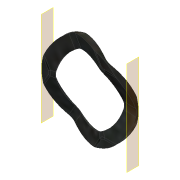
# Autodesk Inventor part: Nema 17 Sprung Washer
Saved by Autodesk Inventor 2020.2 (Build 242310000, 310)
## iProperties
Created: 2020-01-21
Part Number: Nema 17 Sprung Washer
Material: Steel
Document SubType Name: Modeling
Designer: james
Density: 7.85 g/cm^3
Appearance: Plate
Mass: 0.376842 g
Surface Area: 2.38464 cm^2
Volume: 0.0480053 cm^3
Author: james
Autodesk Inventor part; units mm, degrees
ref_plane "XZ Plane" through (0, 0, 0) normal (0, 1, 0) x (-1, 0, 0)
ref_plane "XY Plane" through (0, 0, 0) normal (0, 0, 1) x (1, 0, 0)
sketch "Sketch11" plane through (0, 0, 0) normal (0, 1, 0) x (-1, 0, 0)
  circle A0 centre (0, 0) radius 5.5
  circle A1 centre (0, 0) radius 7.75
  dimension "d82" = 11
  dimension "d83" = 15.5
  constraints: 2 centre point, 2 coincident
  measures "d82" diameter of A0
  measures "d83" diameter of A1
extrude "Extrusion7" add sketch "Sketch11" along normal blind 2
ref_plane "Work Plane6" through (7.75, 0, 0) normal (1, 0, 0) x (0, 1, 0)
sketch "Sketch14" plane through (7.75, 0, 0) normal (1, 0, 0) x (0, 1, 0)
  arc A0 (1.7, 0) -> (1.593716, 0.643303) centre (-0.3, 0) ccw
  line L0 (1.593716, 0.643303) -> (0.053142, 5.178348)
  line L1 (0, -7.75) -> (0, 7.75)
  arc A1 (0, 5.5) -> (0.053142, 5.178348) centre (1, 5.5) ccw
  line L2 (1.7, 0) -> (0, 0)
  line L3 (2, -7.75) -> (2, 7.75) construction
  line L4 (2, -5.5) -> (0, -5.5)
  line L5 (2, 5.5) -> (0, 5.5)
  point P0 (0, 7.75)
  dimension "d100" = 2
  dimension "d101" = 0.3
  dimension "d102" = 1
  constraints: 4 end point, 4 point on circle, 2 centre point, 2 tangent, 1 horizontal, 1 line through centre, 2 other
  measures "d100" radius of A0
  measures "d101" distance from line of L3 L2.start
  measures "d102" radius of A1
extrude "Extrusion10" cut sketch "Sketch14" against normal blind 7.75
mirror "Mirror5" about plane through (0, 0, 0) normal (0, 0, 1) of "Extrusion10"
pattern_circular "Circular Pattern2" count 3 over 360 about axis through (0, 0, 0) along (0, 1, 0) of "Extrusion10", "Mirror5"
ref_plane "Work Plane7" through (-7.75, 0, 0) normal (1, 0, 0) x (0, 1, 0)
sketch "Sketch15" plane through (-7.75, 0, 0) normal (1, 0, 0) x (0, 1, 0)
  line L0 (2, 5.5) -> (2, -5.5)
  line L1 (2, 0) -> (0.3, 0)
  arc A0 (2, -5.5) -> (1.946858, -5.178348) centre (1, -5.5) ccw
  arc A1 (0.3, 0) -> (0.406284, -0.643303) centre (2.3, 0) ccw
  line L2 (1.946858, -5.178348) -> (0.406284, -0.643303)
  point P0 (0, 0)
  dimension "d109" = 1
  dimension "d110" = 2
  dimension "d111" = 0.3
  constraints: 4 end point, 4 point on circle, 3 tangent, 2 centre point, 1 horizontal, 1 line through centre, 1 midpoint
  measures "d109" radius of A0
  measures "d110" radius of A1
  measures "d111" distance of point (0, 0) L1.end
extrude "Extrusion11" cut sketch "Sketch15" along normal blind 7.75
mirror "Mirror6" about plane through (0, 0, 0) normal (0, 0, 1) of "Extrusion11"
pattern_circular "Circular Pattern3" count 3 over 360 about axis through (0, 0, 0) along (0, 1, 0) of "Extrusion11", "Mirror6"
fillet "Fillet8" radius 3 12 edges at (-3.0813, 1.9866, 5.337) (-2.8699, 1.8763, 4.9707) (-2.8699, 1.8763, -4.9707) (-3.0813, 1.9866, -5.337) (6.1626, 1.9866, 0) (5.7397, 1.8763, 0) (2.8699, 0.1237, -4.9707) (3.0813, 0.0134, -5.337) (-6.1626, 0.0134, 0) (-5.7397, 0.1237, 0) (2.8699, 0.1237, 4.9707) (3.0813, 0.0134, 5.337)
body "Solid6"
